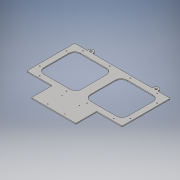
# Autodesk Inventor part: MountPlate
Saved by Autodesk Inventor 2016 (Build 200138000, 138)
## iProperties
Created: 2016-03-06
Part Number: MountPlate
Material: Generic
Document SubType Name: Modeling
Designer: jeffk_000
Density: 1 g/cm^3
Appearance: Default
Author: jeffk_000
Autodesk Inventor part; units mm, degrees
ref_plane "YZ Plane" through (0, 0, 0) normal (1, 0, 0) x (0, 1, 0)
ref_plane "XZ Plane" through (0, 0, 0) normal (0, 1, 0) x (-1, 0, 0)
ref_plane "XY Plane" through (0, 0, 0) normal (0, 0, 1) x (1, 0, 0)
sketch "Sketch1" plane through (0, 0, 0) normal (0, 1, 0) x (-1, 0, 0)
  line L0 (159, -79) -> (-159, -79) construction
  line L1 (-159, -79) -> (-159, 79) construction
  line L2 (-159, 79) -> (159, 79) construction
  line L3 (159, 79) -> (159, -79) construction
  line L4 (153, -73) -> (-153, -73) construction
  line L5 (-153, -73) -> (-153, 73) construction
  line L6 (-153, 73) -> (153, 73) construction
  line L7 (153, 73) -> (153, -73) construction
  circle A0 centre (153, -45) radius 1.6
  circle A1 centre (153, 45) radius 1.6
  circle A2 centre (125, -73) radius 1.6
  circle A3 centre (35, -73) radius 1.6
  circle A4 centre (-35, -73) radius 1.6
  circle A5 centre (-125, -73) radius 1.6
  circle A6 centre (-153, -45) radius 1.6
  circle A7 centre (-153, 45) radius 1.6
  circle A8 centre (125, 73) radius 1.6
  circle A9 centre (35, 73) radius 1.6
  circle A10 centre (-35, 73) radius 1.6
  circle A11 centre (-125, 73) radius 1.6
  line L8 (52.5, 90) -> (-32.5, 90) construction
  line L9 (-32.5, 90) -> (-32.5, 146) construction
  line L10 (-32.5, 146) -> (52.5, 146) construction
  line L11 (52.5, 146) -> (52.5, 90) construction
  circle A12 centre (29, 93.5) radius 1.375
  circle A13 centre (-29, 93.5) radius 1.375
  circle A14 centre (-29, 142.5) radius 1.375
  circle A15 centre (29, 142.5) radius 1.375
  line L12 (104.3189, 118) -> (-116.6862, 118) construction
  circle A16 centre (110, -85) radius 4
  circle A17 centre (-110, -85) radius 4
  arc A18 (101, -85) -> (119, -85) centre (110, -85) ccw
  arc A19 (-119, -85) -> (-101, -85) centre (-110, -85) ccw
  line L13 (99, -81) -> (-99, -81)
  line L14 (101, -83) -> (101, -85)
  line L15 (-101, -83) -> (-101, -85)
  line L16 (159, -81) -> (121, -81)
  line L17 (119, -83) -> (119, -85)
  line L18 (-159, -81) -> (-121, -81)
  line L19 (-119, -83) -> (-119, -85)
  line L20 (161, -79) -> (161, 79)
  line L21 (159, 81) -> (77, 81)
  line L22 (75, 83) -> (75, 149)
  line L23 (73, 151) -> (-73, 151)
  line L24 (-75, 149) -> (-75, 83)
  line L25 (-77, 81) -> (-159, 81)
  line L26 (-161, 79) -> (-161, -79)
  arc A20 (121, -81) -> (119, -83) centre (121, -83) ccw
  arc A21 (159, -81) -> (161, -79) centre (159, -79) ccw
  arc A22 (161, 79) -> (159, 81) centre (159, 79) ccw
  arc A23 (75, 83) -> (77, 81) centre (77, 83) ccw
  arc A24 (75, 149) -> (73, 151) centre (73, 149) ccw
  arc A25 (-73, 151) -> (-75, 149) centre (-73, 149) ccw
  arc A26 (-77, 81) -> (-75, 83) centre (-77, 83) ccw
  arc A27 (-159, 81) -> (-161, 79) centre (-159, 79) ccw
  arc A28 (-161, -79) -> (-159, -81) centre (-159, -79) ccw
  arc A29 (-119, -83) -> (-121, -81) centre (-121, -83) ccw
  arc A30 (-99, -81) -> (-101, -83) centre (-99, -83) ccw
  arc A31 (101, -83) -> (99, -81) centre (99, -83) ccw
  line L27 (122, -62) -> (35, -62)
  line L28 (15, -42) -> (15, 42)
  line L29 (35, 62) -> (122, 62)
  line L30 (142, 42) -> (142, -42)
  line L31 (-35, -62) -> (-122, -62)
  line L32 (-142, -42) -> (-142, 42)
  line L33 (-122, 62) -> (-35, 62)
  line L34 (-15, 42) -> (-15, -42)
  arc A32 (122, -62) -> (142, -42) centre (122, -42) ccw
  arc A33 (142, 42) -> (122, 62) centre (122, 42) ccw
  arc A34 (35, 62) -> (15, 42) centre (35, 42) ccw
  arc A35 (15, -42) -> (35, -62) centre (35, -42) ccw
  arc A36 (-35, -62) -> (-15, -42) centre (-35, -42) ccw
  arc A37 (-142, -42) -> (-122, -62) centre (-122, -42) ccw
  arc A38 (-122, 62) -> (-142, 42) centre (-122, 42) ccw
  arc A39 (-15, 42) -> (-35, 62) centre (-35, 42) ccw
  point P0 (0, 0)
  point P1 (0, -79)
  point P2 (159, 0)
  point P3 (0, -73)
  point P4 (153, 0)
  point P5 (52.5, 118)
  point P6 (75, 151)
  point P7 (-75, 151)
  point P8 (0, 151)
  dimension "d0" = 318
  dimension "d1" = 158
  dimension "d2" = 6
  dimension "d3" = 6
  dimension "d4" = 70
  dimension "d5" = 35
  dimension "d6" = 90
  dimension "d7" = 90
  dimension "d8" = 90
  dimension "d9" = 45
  dimension "d10" = 3.2
  dimension "d11" = 85
  dimension "d12" = 56
  dimension "d13" = 3.5
  dimension "d14" = 2.75
  dimension "d15" = 3.5
  dimension "d16" = 58
  dimension "d17" = 49
  dimension "d18" = 118
  dimension "d19" = 220
  dimension "d20" = 110
  dimension "d21" = 8
  dimension "d22" = 85
  dimension "d23" = 18
  dimension "d24" = 2
  dimension "d25" = 2
  dimension "d26" = 2
  dimension "d27" = 2
  dimension "d28" = 150
  dimension "d29" = 5
  dimension "d30" = 2
  dimension "d31" = 11
  dimension "d32" = 11
  dimension "d33" = 11
  dimension "d34" = 11
  dimension "d35" = 30
  dimension "d36" = 15
  dimension "d37" = 20
  dimension "d40" = 29
  constraints: 70 end point, 44 point on circle, 44 tangent, 40 centre point, 34 equal radius, 17 point on line, 10 parallel, 10 perpendicular, 9 horizontal, 9 vertical alignment, 7 horizontal alignment, 6 midpoint, 6 vertical, 5 collinear, 2 coincident
  measures "d0" distance of L0.start L0.end
  measures "d1" distance of L0.end L1.end
  measures "d2" distance between parallel lines of L4 L0
  measures "d3" distance between parallel lines of L3 L7
  measures "d4" distance of A4.centre A3.centre
  measures "d5" horizontal distance of point (0, 0) A4.centre
  measures "d6" distance of A5.centre A4.centre
  measures "d7" distance of A3.centre A2.centre
  measures "d8" distance of A1.centre A0.centre
  measures "d9" distance of point (153, 0) A0.centre
  measures "d10" diameter of A0
  measures "d11" distance of L9.end L10.end
  measures "d12" distance of L8.end L9.end
  measures "d13" distance from line of L9 A13.centre
  measures "d14" diameter of A13
  measures "d15" distance from line of L8 A13.centre
  measures "d16" distance of A12.centre A13.centre
  measures "d17" distance of A14.centre A13.centre
  measures "d18" distance from line of L12 point (0, 0)
  measures "d19" distance of A17.centre A16.centre
  measures "d20" horizontal distance of point (0, 0) A17.centre
  measures "d21" diameter of A17
  measures "d22" vertical distance of A16.centre point (0, 0)
  measures "d23" diameter of A18
  measures "d24" distance between parallel lines of L13 L0
  measures "d25" distance between parallel lines of L26 L1
  measures "d26" distance between parallel lines of L3 L20
  measures "d27" distance between parallel lines of L2 L21
  measures "d28" distance of point (75, 151) point (-75, 151)
  measures "d29" distance between parallel lines of L23 L10
  measures "d30" radius of A20
  measures "d31" distance between parallel lines of L5 L32
  measures "d32" distance between parallel lines of L7 L30
  measures "d33" distance between parallel lines of L29 L6
  measures "d34" distance between parallel lines of L27 L4
  measures "d35" distance between parallel lines of L34 L28
  measures "d36" distance from line of point (0, 0) L34
  measures "d37" radius of A32
  measures "d40" horizontal distance of point (0, 0) A12.centre
extrude "Extrusion1" add sketch "Sketch1" along normal blind 3
sketch "Sketch2" plane through (0, 3, 0) normal (0, 1, 0) x (1, 0, 0)
  arc A0 (142, 42) -> (122, 62) centre (122, 42) ccw projected
  line L0 (142, 42) -> (142, -42) projected
  arc A1 (122, -62) -> (142, -42) centre (122, -42) ccw projected
  line L1 (122, -62) -> (35, -62) projected
  arc A2 (15, -42) -> (35, -62) centre (35, -42) ccw projected
  line L2 (15, -42) -> (15, 42) projected
  arc A3 (35, 62) -> (15, 42) centre (35, 42) ccw projected
  line L3 (35, 62) -> (122, 62) projected
  arc A4 (-122, 62) -> (-142, 42) centre (-122, 42) ccw projected
  line L4 (-122, 62) -> (-35, 62) projected
  arc A5 (-15, 42) -> (-35, 62) centre (-35, 42) ccw projected
  line L5 (-15, 42) -> (-15, -42) projected
  arc A6 (-35, -62) -> (-15, -42) centre (-35, -42) ccw projected
  line L6 (-35, -62) -> (-122, -62) projected
  arc A7 (-142, -42) -> (-122, -62) centre (-122, -42) ccw projected
  line L7 (-142, -42) -> (-142, 42) projected
  circle A8 centre (110, 85) radius 4 projected
  circle A9 centre (-110, 85) radius 4 projected
  circle A10 centre (125, -73) radius 1.6 projected
  circle A11 centre (35, -73) radius 1.6 projected
  circle A12 centre (-35, -73) radius 1.6 projected
  circle A13 centre (-125, -73) radius 1.6 projected
  circle A14 centre (153, -45) radius 1.6 projected
  circle A15 centre (153, 45) radius 1.6 projected
  circle A16 centre (125, 73) radius 1.6 projected
  circle A17 centre (35, 73) radius 1.6 projected
  circle A18 centre (-35, 73) radius 1.6 projected
  circle A19 centre (-125, 73) radius 1.6 projected
  circle A20 centre (-153, -45) radius 1.6 projected
  circle A21 centre (-153, 45) radius 1.6 projected
  circle A22 centre (-29, -142.5) radius 1.375 projected
  circle A23 centre (29, -142.5) radius 1.375 projected
  circle A24 centre (29, -93.5) radius 1.375 projected
  circle A25 centre (-29, -93.5) radius 1.375 projected
  line L8 (-101, 83) -> (-101, 85) projected
  arc A26 (-101, 85) -> (-119, 85) centre (-110, 85) ccw projected
  line L9 (-119, 85) -> (-119, 83) projected
  arc A27 (-121, 81) -> (-119, 83) centre (-121, 83) ccw projected
  line L10 (-121, 81) -> (-159, 81) projected
  arc A28 (-159, 81) -> (-161, 79) centre (-159, 79) ccw projected
  line L11 (-161, 79) -> (-161, -79) projected
  arc A29 (-161, -79) -> (-159, -81) centre (-159, -79) ccw projected
  line L12 (-159, -81) -> (-77, -81) projected
  arc A30 (-75, -83) -> (-77, -81) centre (-77, -83) ccw projected
  line L13 (-75, -83) -> (-75, -149) projected
  arc A31 (-75, -149) -> (-73, -151) centre (-73, -149) ccw projected
  line L14 (-73, -151) -> (73, -151) projected
  arc A32 (73, -151) -> (75, -149) centre (73, -149) ccw projected
  line L15 (75, -149) -> (75, -83) projected
  arc A33 (77, -81) -> (75, -83) centre (77, -83) ccw projected
  line L16 (77, -81) -> (159, -81) projected
  arc A34 (159, -81) -> (161, -79) centre (159, -79) ccw projected
  line L17 (161, -79) -> (161, 79) projected
  arc A35 (161, 79) -> (159, 81) centre (159, 79) ccw projected
  line L18 (159, 81) -> (121, 81) projected
  arc A36 (119, 83) -> (121, 81) centre (121, 83) ccw projected
  line L19 (119, 83) -> (119, 85) projected
  arc A37 (119, 85) -> (101, 85) centre (110, 85) ccw projected
  line L20 (101, 85) -> (101, 83) projected
  arc A38 (99, 81) -> (101, 83) centre (99, 83) ccw projected
  line L21 (99, 81) -> (-99, 81) projected
  arc A39 (-101, 83) -> (-99, 81) centre (-99, 83) ccw projected
  line L22 (-99, 81.1) -> (99, 81.1)
  arc A40 (99, 81.1) -> (100.9, 83) centre (99, 83) ccw
  line L23 (100.9, 83) -> (100.9, 85)
  arc A41 (119.1, 85) -> (100.9, 85) centre (110, 85) ccw
  line L24 (119.1, 85) -> (119.1, 83)
  arc A42 (119.1, 83) -> (121, 81.1) centre (121, 83) ccw
  line L25 (121, 81.1) -> (159, 81.1)
  arc A43 (161.1, 79) -> (159, 81.1) centre (159, 79) ccw
  line L26 (161.1, 79) -> (161.1, -79)
  arc A44 (159, -81.1) -> (161.1, -79) centre (159, -79) ccw
  line L27 (159, -81.1) -> (77, -81.1)
  arc A45 (77, -81.1) -> (75.1, -83) centre (77, -83) ccw
  line L28 (75.1, -83) -> (75.1, -149)
  arc A46 (73, -151.1) -> (75.1, -149) centre (73, -149) ccw
  line L29 (73, -151.1) -> (-73, -151.1)
  arc A47 (-75.1, -149) -> (-73, -151.1) centre (-73, -149) ccw
  line L30 (-75.1, -149) -> (-75.1, -83)
  arc A48 (-75.1, -83) -> (-77, -81.1) centre (-77, -83) ccw
  line L31 (-77, -81.1) -> (-159, -81.1)
  arc A49 (-161.1, -79) -> (-159, -81.1) centre (-159, -79) ccw
  line L32 (-161.1, -79) -> (-161.1, 79)
  arc A50 (-159, 81.1) -> (-161.1, 79) centre (-159, 79) ccw
  line L33 (-159, 81.1) -> (-121, 81.1)
  arc A51 (-121, 81.1) -> (-119.1, 83) centre (-121, 83) ccw
  line L34 (-119.1, 83) -> (-119.1, 85)
  arc A52 (-100.9, 85) -> (-119.1, 85) centre (-110, 85) ccw
  line L35 (-100.9, 85) -> (-100.9, 83)
  arc A53 (-100.9, 83) -> (-99, 81.1) centre (-99, 83) ccw
  line L36 (-35, 61.9) -> (-122, 61.9)
  arc A54 (-122, 61.9) -> (-141.9, 42) centre (-122, 42) ccw
  line L37 (-141.9, 42) -> (-141.9, -42)
  arc A55 (-141.9, -42) -> (-122, -61.9) centre (-122, -42) ccw
  line L38 (-122, -61.9) -> (-35, -61.9)
  arc A56 (-35, -61.9) -> (-15.1, -42) centre (-35, -42) ccw
  line L39 (-15.1, -42) -> (-15.1, 42)
  arc A57 (-15.1, 42) -> (-35, 61.9) centre (-35, 42) ccw
  arc A58 (141.9, 42) -> (122, 61.9) centre (122, 42) ccw
  line L40 (141.9, 42) -> (141.9, -42)
  arc A59 (122, -61.9) -> (141.9, -42) centre (122, -42) ccw
  line L41 (122, -61.9) -> (35, -61.9)
  arc A60 (15.1, -42) -> (35, -61.9) centre (35, -42) ccw
  line L42 (15.1, -42) -> (15.1, 42)
  arc A61 (35, 61.9) -> (15.1, 42) centre (35, 42) ccw
  line L43 (35, 61.9) -> (122, 61.9)
  circle A62 centre (-110, 85) radius 3.9
  circle A63 centre (110, 85) radius 3.9
  circle A64 centre (35, 73) radius 1.5
  circle A65 centre (-35, 73) radius 1.5
  circle A66 centre (-125, 73) radius 1.5
  circle A67 centre (-153, 45) radius 1.5
  circle A68 centre (-153, -45) radius 1.5
  circle A69 centre (-125, -73) radius 1.5
  circle A70 centre (-35, -73) radius 1.5
  circle A71 centre (35, -73) radius 1.5
  circle A72 centre (125, -73) radius 1.5
  circle A73 centre (153, -45) radius 1.5
  circle A74 centre (153, 45) radius 1.5
  circle A75 centre (125, 73) radius 1.5
  circle A76 centre (-29, -93.5) radius 1.275
  circle A77 centre (29, -93.5) radius 1.275
  circle A78 centre (29, -142.5) radius 1.275
  circle A79 centre (-29, -142.5) radius 1.275
  circle A80 centre (125, -73) radius 1.6 projected
  point P0 (0, 0)
  dimension "d41" = 0.1
  dimension "d42" = 0.1
  dimension "d43" = 0.1
  dimension "d44" = 0.1
  dimension "d45" = 0.1
  dimension "d46" = 0.1
  dimension "d47" = 0.1
  dimension "d48" = 0.1
  dimension "d49" = 0.1
  dimension "d50" = 0.1
  dimension "d51" = 0.1
  dimension "d52" = 0.1
  dimension "d54" = 0.1
  dimension "d55" = 0.1
  dimension "d56" = 0.1
  dimension "d57" = 0.1
  dimension "d58" = 0.1
  dimension "d59" = 0.1
  dimension "d60" = 0.1
  dimension "d61" = 0.1
  dimension "d62" = 0.1
  constraints: 44 end point, 44 point on circle, 40 centre point, 41 other
  measures "d41" distance between parallel lines of L21 L22
  measures "d42" distance between parallel lines of L36 L4
  measures "d43" distance between parallel lines of L3 L43
  measures "d44" radial gap between concentric circles of A9 A62
  measures "d45" radial gap between concentric circles of A8 A63
  measures "d46" radial gap between concentric circles of A66 A19
  measures "d47" radial gap between concentric circles of A18 A65
  measures "d48" radial gap between concentric circles of A17 A64
  measures "d49" radial gap between concentric circles of A16 A75
  measures "d50" radial gap between concentric circles of A21 A67
  measures "d51" radial gap between concentric circles of A20 A68
  measures "d52" radial gap between concentric circles of A13 A69
  measures "d54" radial gap between concentric circles of A12 A70
  measures "d55" radial gap between concentric circles of A11 A71
  measures "d56" radial gap between concentric circles of A80 A72
  measures "d57" radial gap between concentric circles of A14 A73
  measures "d58" radial gap between concentric circles of A15 A74
  measures "d59" radial gap between concentric circles of A25 A76
  measures "d60" radial gap between concentric circles of A24 A77
  measures "d61" radial gap between concentric circles of A23 A78
  measures "d62" radial gap between concentric circles of A22 A79
extrude "Extrusion2" add sketch "Sketch2" against normal blind 3
equation "\"d5\" = 0.5 * d4"
equation "\"d7\" = d6"
equation "\"d9\" = 0.5 * d8"
equation "\"d20\" = 0.5 * d19"
equation "\"d25\" = d24"
equation "\"d26\" = d25"
equation "\"d27\" = d24"
equation "\"d32\" = d31"
equation "\"d33\" = d31"
equation "\"d34\" = d31"
equation "\"d36\" = 0.5 * d35"
equation "\"d40\" = 0.5 * d16"
equation "\"d41\" = 0.5 * kerf"
equation "\"d42\" = 0.5 * kerf"
equation "\"d43\" = 0.5 * kerf"
equation "\"d44\" = 0.5 * kerf"
equation "\"d45\" = 0.5 * kerf"
equation "\"d46\" = 0.5 * kerf"
equation "\"d47\" = 0.5 * kerf"
equation "\"d48\" = 0.5 * kerf"
equation "\"d49\" = 0.5 * kerf"
equation "\"d50\" = 0.5 * kerf"
equation "\"d51\" = 0.5 * kerf"
equation "\"d52\" = 0.5 * kerf"
equation "\"d54\" = 0.5 * kerf"
equation "\"d55\" = 0.5 * kerf"
equation "\"d56\" = 0.5 * kerf"
equation "\"d57\" = 0.5 * kerf"
equation "\"d58\" = 0.5 * kerf"
equation "\"d59\" = 0.5 * kerf"
equation "\"d60\" = 0.5 * kerf"
equation "\"d61\" = 0.5 * kerf"
equation "\"d62\" = 0.5 * kerf"
equation "\"kerf\" = 0.2"
body "Solid1"
